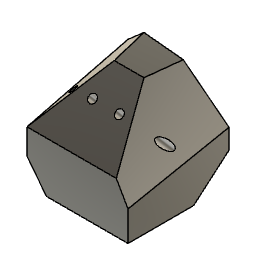
Suètone-drawing-object-01 v2 (Autodesk Fusion 360 design; units mm, degrees)
Autodesk Fusion 360 part; units mm, degrees
sketch "Esquisse1" plane through (0, 0, 0) normal (0, 0, 1) x (1, 0, 0)
  line L0 (50, 50) -> (-50, 50)
  line L1 (-50, 50) -> (-50, -50)
  line L2 (-50, -50) -> (50, -50)
  line L3 (50, -50) -> (50, 50)
  line L4 (50, 50) -> (-50, -50) construction
  line L5 (-50, 50) -> (50, -50) construction
  dimension "d1" = 100
  dimension "d2" = 100
  constraint horizontal L0
  constraint perpendicular L0 L1
  constraint parallel L0 L2
  constraint parallel L1 L3
  constraint coincident L4 origin
  constraint coincident L5 origin
  measures "d1" distance of L1.end L2.end
  measures "d2" distance of L0.end L1.end
extrude "Extrusion1" add sketch "Esquisse1" along normal blind 100 makes body 1
sketch "Esquisse2" plane through (50, 0, 0) normal (1, 0, 0) x (0, 1, 0)
  line L0 (-50, 0) -> (50, 0)
  line L1 (50, 0) -> (50, 100)
  line L2 (50, 100) -> (-50, 100)
  line L3 (-50, 100) -> (-50, 0)
  line L4 (-50, 50) -> (50, 70)
  constraint midpoint L3 L4.start
  constraint coincident L1 L4.end
ref_plane "Plan de construction2" through (50, 0, 60) normal (0.866025, -0.098058, 0.49029) x (0, 0.980581, 0.196116)
split "Scinder1" by plane through (50, 0, 60) normal (0.866025, -0.098058, 0.49029) bodies 1 makes body 2 at (50, -16.6667, 73.3333)
delete_body "RemoveBody1" bodies 2
sketch "Esquisse3" plane through (0, -50, 0) normal (0, -1, 0) x (1, 0, 0)
  line L0 (50, 50) -> (21.6931, 100)
  line L1 (21.6931, 100) -> (-50, 100)
  line L2 (-50, 100) -> (-50, 0)
  line L3 (-50, 0) -> (50, 0)
  line L4 (50, 0) -> (50, 50)
  line L5 (50, 50) -> (-50, 50)
  constraint coincident L0.start L4.end
  constraint midpoint L2 L5.end
ref_plane "Plan de construction3" through (0, -50, 50) normal (0, -0.707107, 0.707107) x (-1, 0, 0)
split "Scinder2" by plane through (0, -50, 50) normal (0, -0.707107, 0.707107) bodies 1 makes body 3 at (7.231, -50, 66.6667)
delete_body "RemoveBody2" bodies 3
sketch "Esquisse4" plane through (-50, 0, 0) normal (-1, 0, 0) x (0, -1, 0)
  line L0 (50, 50) -> (0, 100)
  line L1 (0, 100) -> (-50, 100)
  line L2 (-50, 100) -> (-50, 0)
  line L3 (-50, 0) -> (50, 0)
  line L4 (50, 0) -> (50, 50)
  line L5 (50, 50) -> (-50, 75)
  constraint coincident L0.start L4.end
  constraint coincident L2 L5.end
ref_plane "Plan de construction4" through (-50, 0, 62.5) normal (0.707107, 0.171499, -0.685994) x (0, 0.970143, 0.242536)
split "Scinder3" by plane through (-50, 0, 62.5) normal (0.707107, 0.171499, -0.685994) bodies 1 makes body 4 at (-16.6667, 16.6667, 0)
delete_body "RemoveBody3" bodies 1
sketch "Esquisse5" plane through (-50, 0, 0) normal (-1, 0, 0) x (0, -1, 0)
  line L0 (50, 50) -> (-50, 75)
  line L1 (-50, 75) -> (-50, 0)
  line L2 (-50, 0) -> (50, 0)
  line L3 (50, 0) -> (50, 50)
  line L4 (50, 25) -> (20, 0)
  constraint midpoint L3 L4.start
  constraint coincident L2 L4.end
ref_plane "Plan de construction5" through (-50, -35, 12.5) normal (0.707107, 0.452679, 0.543214) x (0, 0.768221, -0.640184)
split "Scinder4" by plane through (-50, -35, 12.5) normal (0.707107, 0.452679, 0.543214) bodies 4 makes body 5 at (16.6667, -6.6667, 0)
delete_body "RemoveBody4" bodies 4
sketch "Esquisse6" plane through (50, 0, 0) normal (1, 0, 0) x (0, 1, 0)
  line L0 (50, 70) -> (-50, 50)
  line L1 (-50, 50) -> (-50, 0)
  line L2 (-50, 0) -> (50, 0)
  line L3 (50, 0) -> (50, 70)
  line L4 (50, 30) -> (15, 0)
  constraint coincident L3 L4.start
  constraint coincident L2 L4.end
ref_plane "Plan de construction6" through (50, 32.5, 15) normal (0, -0.650791, 0.759257) x (0, -0.759257, -0.650791)
split "Scinder5" by plane through (50, 32.5, 15) normal (0, -0.650791, 0.759257) bodies 5 makes body 6 at (-8.5821, 50, 66.6667)
delete_body "RemoveBody5" bodies 5
sketch "Esquisse7" plane through (0, 6.3529, -7.4118) normal (0, 0.650791, -0.759257) x (-1, 0, 0)
  line L0 (-50, 11.3888) -> (50, 11.3888)
  line L1 (50, 11.3888) -> (50, 57.4866)
  line L2 (50, 57.4866) -> (-50, 57.4866)
  line L3 (-50, 57.4866) -> (-50, 11.3888)
  circle A0 centre (-39.8919, 34.4377) radius 4
  circle A1 centre (-13.2252, 34.4377) radius 4
  circle A2 centre (13.4414, 34.4377) radius 4
  circle A3 centre (40.1081, 34.4377) radius 4
  dimension "d11" = 8
  dimension "d14" = 80
  dimension "d15" = 0
  measures "d11" diameter of A0
move_face "DécalerLesFaces1" offset -10 1 faces at (42.4515, 0, 73.3333) on bodies 6
extrude "Extrusion2" cut sketch "Esquisse7" against normal blind 90 contours A0 | A1 | A2 | A3 bodies 6
sketch "Esquisse8" plane through (0, 0, 0) normal (0, 0, -1) x (1, 0, 0)
  line L0 (-50, -15) -> (50, -15)
  line L1 (50, -15) -> (50, 50)
  line L2 (50, 50) -> (-30.7945, 50)
  line L3 (-30.7945, 50) -> (-50, 20)
  line L4 (-50, 20) -> (-50, -15)
  line L5 (-25.9096, 44.0764) -> (44.0904, 44.0764)
  line L6 (44.0904, 44.0764) -> (44.0904, 40.0764)
  line L7 (44.0904, 40.0764) -> (-25.9096, 40.0764)
  line L8 (-25.9096, 40.0764) -> (-25.9096, 44.0764)
  line L9 (-45, -10) -> (45, -10)
  line L10 (45, -10) -> (45, -6)
  line L11 (45, -6) -> (-45, -6)
  line L12 (-45, -6) -> (-45, -10)
  dimension "d19" = 70
  dimension "d20" = 4
  dimension "d21" = 90
  dimension "d22" = 4
  constraint horizontal L5
  constraint vertical L6
  constraint horizontal L7
  constraint vertical L8
  constraint horizontal L9
  constraint vertical L10
  constraint horizontal L11
  constraint vertical L12
  measures "d19" distance of L5.start L5.end
  measures "d20" distance of L5.start L7.end
  measures "d21" distance of L9.start L9.end
  measures "d22" distance of L9.start L11.end
extrude "Extrusion4" add sketch "Esquisse8" along normal blind 2 separate body contours L5 L6 L7 L8 | L9 L10 L11 L12 makes body 7 at (-15, 7.3333, 0) makes body 8 at (-2.5762, -42.743, 0)
sketch "Esquisse9" plane through (0, 50, 0) normal (0, 1, 0) x (-1, 0, 0)
  line L0 (-50, 30) -> (50, 30)
  line L1 (50, 30) -> (50, 75)
  line L2 (50, 75) -> (25.7464, 100)
  line L3 (25.7464, 100) -> (-21.4688, 100)
  line L4 (-21.4688, 100) -> (-50, 49.6039)
  line L5 (-50, 49.6039) -> (-50, 30)
  line L6 (-50, 49.6039) -> (50, 75)
  constraint coincident L4.end L5.start
  constraint coincident L1.end L2.start
ref_plane "Plan de construction7" through (0, 50, 62.302) normal (0.084187, 0.939693, 0.331497) x (-0.969232, 0, 0.246147)
split "Scinder6" by plane through (0, 50, 62.302) normal (0.084187, 0.939693, 0.331497) bodies 6 makes body 9 at (-8.5821, 50, 74.868)
delete_body "RemoveBody6" bodies 9
